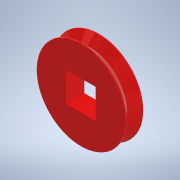
# Autodesk Inventor part: pulley
Saved by Autodesk Inventor 2020 (Build 240168000, 168)
## iProperties
Created: 2020-02-03
Part Number: pulley
Material: PC/ABS Plastic
Document SubType Name: Modeling
Designer: Felix
Density: 0.357273 g/cm^3
Appearance: Smooth - Red
Author: Felix
Autodesk Inventor part; units mm, degrees
ref_plane "YZ Plane" through (0, 0, 0) normal (1, 0, 0) x (0, 1, 0)
ref_plane "XZ Plane" through (0, 0, 0) normal (0, 1, 0) x (-1, 0, 0)
ref_plane "XY Plane" through (0, 0, 0) normal (0, 0, 1) x (1, 0, 0)
sketch "Sketch1" plane through (0, 0, 0) normal (1, 0, 0) x (0, 1, 0)
  line L0 (0, 0) -> (0, 2)
  line L1 (0, 1) -> (4, 1) construction
  line L2 (5, 2) -> (4, 1)
  line L3 (4, 1) -> (5, 0)
  line L4 (5, 2) -> (0, 2)
  line L5 (5, 0) -> (0, 0)
  dimension "d0" = 2
  dimension "d2" = 1
  dimension "d3" = 1
  dimension "d4" = 1
  dimension "d5" = 5
  constraints: 12 end point, 1 horizontal, 1 midpoint, 1 parallel, 1 perpendicular, 1 vertical
  measures "d0" distance of L0.start L0.end
  measures "d2" distance from line of L4 L1.end
  measures "d3" horizontal distance of L2.start L1.end
  measures "d4" horizontal distance of L1.end L3.end
  measures "d5" distance of L0.end L2.start
revolve "Revolution1" add sketch "Sketch1" angle 360 about axis through (0, 0, 0) along (0, 0, 1)
fillet "Fillet1" radius 0.1 2 edges at (0, -5, 2) (0, -5, 0)
sketch "Sketch2" plane through (0, 0, 2) normal (0, 0, 1) x (1, 0, 0)
  circle A0 centre (0, 0) radius 4 construction
  line L0 (-1.6, 1.6) -> (1.6, 1.6)
  line L1 (1.6, 1.6) -> (1.6, -1.6)
  line L2 (1.6, -1.6) -> (-1.6, -1.6)
  line L3 (-1.6, -1.6) -> (-1.6, 1.6)
  line L4 (-1.6, 1.6) -> (1.6, -1.6) construction
  line L5 (1.6, 1.6) -> (-1.6, -1.6) construction
  dimension "d8" = 3.2
  dimension "d9" = 3.2
  constraints: 12 end point, 2 midpoint, 2 parallel, 1 horizontal, 1 perpendicular
  measures "d8" distance of L1.end L2.end
  measures "d9" distance of L0.end L1.end
extrude "Extrusion1" cut sketch "Sketch2" against normal through all
equation "\"d3\" = d2"
equation "\"d4\" = d3"
equation "\"d9\" = d8"
body "Solid1"
